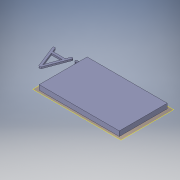
# Autodesk Inventor part: stamp5x3
Saved by Autodesk Inventor 2019 (Build 230136000, 136)
## iProperties
Created: 2019-02-19
Part Number: stamp5x3
Material: PET Plastic
Document SubType Name: Modeling
Designer: jmc
Density: 1.541 g/cm^3
Appearance: Slate Blue
Author: jmc
Autodesk Inventor part; units mm, degrees
ref_plane "YZ Plane" through (0, 0, 0) normal (1, 0, 0) x (0, 1, 0)
ref_plane "XZ Plane" through (0, 0, 0) normal (0, 1, 0) x (-1, 0, 0)
ref_plane "XY Plane" through (0, 0, 0) normal (0, 0, 1) x (1, 0, 0)
sketch "Sketch1" plane through (0, 0, 0) normal (0, 1, 0) x (-1, 0, 0)
  line L0 (24.925, 14.925) -> (-24.925, 14.925)
  line L1 (-24.925, 14.925) -> (-24.925, -14.925)
  line L2 (-24.925, -14.925) -> (24.925, -14.925)
  line L3 (24.925, 14.925) -> (-24.925, -14.925) construction
  line L4 (-24.925, 14.925) -> (24.925, -14.925) construction
  line L5 (24.925, -14.925) -> (24.925, 14.925)
  line L6 (24.925, 5) -> (24.925, 14.925)
  point P0 (0, 0)
  dimension "d0" = 49.85
  dimension "d1" = 29.85
  constraints: 14 end point, 3 parallel, 2 midpoint, 1 horizontal, 1 perpendicular
  measures "d0" distance of L2.end L1.end
  measures "d1" distance of L1.end L0.end
extrude "Extrusion1" add sketch "Sketch1" along normal blind 3
sketch "Sketch2" plane through (0, 0, 0) normal (0, -1, 0) x (1, 0, 0)
  point P0 (0, 0)
sketch "Sketch3" plane through (-24.925, 0, -14.925) normal (-1, 0, 0) x (0, 0, 1)
  point P0 (14.925, 0)
ref_plane "Work Plane1" through (0, 0, 0) normal (0, 1, 0) x (-1, 0, 0)
sketch "Sketch5" plane through (0, 0, 0) normal (0, 1, 0) x (-1, 0, 0)
  line L0 (-8.9097, 2.0147) -> (44.6537, 2.0147) construction
  line L1 (44.6537, 2.0147) -> (44.6537, -13.1558) construction
  line L2 (44.6537, -13.1558) -> (-8.9097, -13.1558) construction
  line L3 (-8.9097, -13.1558) -> (-8.9097, 2.0147) construction
  spline S0 degree 2 poles (2.4399, -12.3712) (2.4399, -13.0649) (1.7916, -13.0649) knots 0 0 0 1 1 1
  spline S1 degree 2 poles (1.7916, -13.0649) (1.132, -13.0649) (1.132, -12.3712) knots 0 0 0 1 1 1
  line L4 (1.132, -12.3712) -> (1.132, -5.8662)
  line L5 (1.132, -5.8662) -> (-6.3964, -5.8662)
  line L6 (-6.3964, -5.8662) -> (-6.3964, -12.3712)
  spline S2 degree 2 poles (-6.3964, -12.3712) (-6.3964, -13.0649) (-7.056, -13.0649) knots 0 0 0 1 1 1
  spline S3 degree 2 poles (-7.056, -13.0649) (-7.7269, -13.0649) (-7.7269, -12.3712) knots 0 0 0 1 1 1
  line L7 (-7.7269, -12.3712) -> (-7.7269, 1.1959)
  spline S4 degree 2 poles (-7.7269, 1.1959) (-7.7269, 1.8896) (-7.056, 1.8896) knots 0 0 0 1 1 1
  spline S5 degree 2 poles (-7.056, 1.8896) (-6.3964, 1.8896) (-6.3964, 1.1959) knots 0 0 0 1 1 1
  line L8 (-6.3964, 1.1959) -> (-6.3964, -4.4902)
  line L9 (-6.3964, -4.4902) -> (1.132, -4.4902)
  line L10 (1.132, -4.4902) -> (1.132, 1.1959)
  spline S6 degree 2 poles (1.132, 1.1959) (1.132, 1.8896) (1.7916, 1.8896) knots 0 0 0 1 1 1
  spline S7 degree 2 poles (1.7916, 1.8896) (2.4399, 1.8896) (2.4399, 1.1959) knots 0 0 0 1 1 1
  line L11 (2.4399, 1.1959) -> (2.4399, -12.3712)
  spline S8 degree 2 poles (17.1783, -5.6502) (17.1783, -8.6979) (15.7454, -10.8245) knots 0 0 0 1 1 1
  spline S9 degree 2 poles (15.7454, -10.8245) (14.176, -13.1558) (11.6286, -13.1558) knots 0 0 0 1 1 1
  spline S10 degree 2 poles (11.6286, -13.1558) (9.104, -13.1558) (7.4891, -10.8245) knots 0 0 0 1 1 1
  spline S11 degree 2 poles (7.4891, -10.8245) (5.988, -8.6524) (5.988, -5.6502) knots 0 0 0 1 1 1
  spline S12 degree 2 poles (5.988, -5.6502) (5.988, -2.6251) (7.3982, -0.3962) knots 0 0 0 1 1 1
  spline S13 degree 2 poles (7.3982, -0.3962) (8.9448, 2.0147) (11.3898, 2.0147) knots 0 0 0 1 1 1
  spline S14 degree 2 poles (11.3898, 2.0147) (14.0054, 2.0147) (15.6544, -0.3962) knots 0 0 0 1 1 1
  spline S15 degree 2 poles (15.6544, -0.3962) (17.1783, -2.6251) (17.1783, -5.6502) knots 0 0 0 1 1 1
  spline S16 degree 2 poles (15.8477, -5.6502) (15.8477, -3.1255) (14.7333, -1.3628) knots 0 0 0 1 1 1
  spline S17 degree 2 poles (14.7333, -1.3628) (13.4937, 0.6387) (11.3898, 0.6387) knots 0 0 0 1 1 1
  spline S18 degree 2 poles (11.3898, 0.6387) (9.4338, 0.6387) (8.3193, -1.3628) knots 0 0 0 1 1 1
  spline S19 degree 2 poles (8.3193, -1.3628) (7.3413, -3.1028) (7.3413, -5.6502) knots 0 0 0 1 1 1
  spline S20 degree 2 poles (7.3413, -5.6502) (7.3413, -8.152) (8.4103, -9.892) knots 0 0 0 1 1 1
  spline S21 degree 2 poles (8.4103, -9.892) (9.6044, -11.8025) (11.6286, -11.8025) knots 0 0 0 1 1 1
  spline S22 degree 2 poles (11.6286, -11.8025) (13.6756, -11.8025) (14.8242, -9.892) knots 0 0 0 1 1 1
  spline S23 degree 2 poles (14.8242, -9.892) (15.8477, -8.1748) (15.8477, -5.6502) knots 0 0 0 1 1 1
  line L12 (28.9713, -12.8715) -> (19.8508, -12.8715)
  line L13 (19.8508, -12.8715) -> (19.8508, 1.1959)
  spline S24 degree 2 poles (19.8508, 1.1959) (19.8508, 1.8896) (20.5217, 1.8896) knots 0 0 0 1 1 1
  spline S25 degree 2 poles (20.5217, 1.8896) (21.1813, 1.8896) (21.1813, 1.1959) knots 0 0 0 1 1 1
  line L14 (21.1813, 1.1959) -> (21.1813, -11.5182)
  line L15 (21.1813, -11.5182) -> (28.9713, -11.5182)
  spline S26 degree 2 poles (28.9713, -11.5182) (29.6423, -11.5182) (29.6423, -12.1892) knots 0 0 0 1 1 1
  spline S27 degree 2 poles (29.6423, -12.1892) (29.6423, -12.8715) (28.9713, -12.8715) knots 0 0 0 1 1 1
  spline S28 degree 2 poles (43.8007, -12.1778) (43.8576, -12.3029) (43.8576, -12.4621) knots 0 0 0 1 1 1
  spline S29 degree 2 poles (43.8576, -12.4621) (43.8576, -13.0876) (43.1753, -13.0876) knots 0 0 0 1 1 1
  spline S30 degree 2 poles (43.1753, -13.0876) (42.7431, -13.0876) (42.5612, -12.6555) knots 0 0 0 1 1 1
  line L16 (42.5612, -12.6555) -> (41.5831, -10.1991)
  line L17 (41.5831, -10.1991) -> (33.7704, -10.1991)
  line L18 (33.7704, -10.1991) -> (32.8265, -12.6555)
  spline S31 degree 2 poles (32.8265, -12.6555) (32.6559, -13.0876) (32.2124, -13.0876) knots 0 0 0 1 1 1
  spline S32 degree 2 poles (32.2124, -13.0876) (31.5414, -13.0876) (31.5414, -12.4394) knots 0 0 0 1 1 1
  spline S33 degree 2 poles (31.5414, -12.4394) (31.5414, -12.3029) (31.5869, -12.1778) knots 0 0 0 1 1 1
  line L19 (31.5869, -12.1778) -> (36.7045, 1.4461)
  spline S34 degree 2 poles (36.7045, 1.4461) (36.9205, 2.0147) (37.5687, 2.0147) knots 0 0 0 1 1 1
  spline S35 degree 2 poles (37.5687, 2.0147) (38.2511, 2.0147) (38.4672, 1.4461) knots 0 0 0 1 1 1
  line L20 (38.4672, 1.4461) -> (43.8007, -12.1778)
  line L21 (41.06, -8.823) -> (37.5687, 0.036)
  line L22 (37.5687, 0.036) -> (34.2935, -8.823)
  line L23 (34.2935, -8.823) -> (41.06, -8.823)
  point P0 (0, 0)
  constraints: 2 other
extrude "Extrusion3" add sketch "Sketch5" against normal blind 1
body "Solid1"
